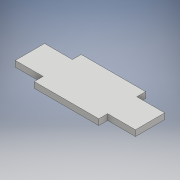
# Autodesk Inventor part: Game_TurmoilTerraformerReplacement
Saved by Autodesk Inventor 2018 (Build 220112000, 112)
## iProperties
Created: 2021-04-21
Part Number: Game_TurmoilTerraformerReplacement
Material: Generic
Document SubType Name: Modeling
Designer: Bradley
Density: 1 g/cm^3
Appearance: Default
Author: Bradley
Autodesk Inventor part; units mm, degrees
ref_plane "YZ Plane" through (0, 0, 0) normal (1, 0, 0) x (0, 1, 0)
ref_plane "XZ Plane" through (0, 0, 0) normal (0, 1, 0) x (-1, 0, 0)
ref_plane "XY Plane" through (0, 0, 0) normal (0, 0, 1) x (1, 0, 0)
sketch "Sketch1" plane through (0, 0, 0) normal (0, 0, 1) x (1, 0, 0)
  line L0 (-20.5, -5) -> (20.5, -5)
  line L1 (20.5, -5) -> (20.5, 5)
  line L2 (20.5, 5) -> (-20.5, 5)
  line L3 (-20.5, 5) -> (-20.5, -5)
  line L4 (-20.5, -5) -> (20.5, 5) construction
  line L5 (20.5, -5) -> (-20.5, 5) construction
  line L6 (-11, -8) -> (11, -8)
  line L7 (11, -8) -> (11, 8)
  line L8 (11, 8) -> (-11, 8)
  line L9 (-11, 8) -> (-11, -8)
  line L10 (-11, -8) -> (11, 8) construction
  line L11 (11, -8) -> (-11, 8) construction
  point P0 (0, 0)
  dimension "d0" = 41
  dimension "d1" = 10
  dimension "d2" = 22
  dimension "d3" = 16
  constraints: 24 end point, 4 midpoint, 4 parallel, 2 horizontal, 2 perpendicular
  measures "d0" distance of L2.end L1.end
  measures "d1" distance of L1.end L0.end
  measures "d2" distance of L8.end L7.end
  measures "d3" distance of L7.end L6.end
extrude "Extrusion1" add sketch "Sketch1" along normal mid plane 2
body "Solid1"
